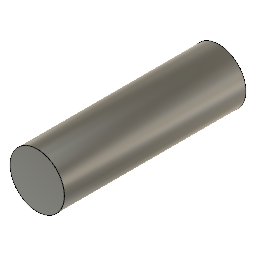
stone_holder (Autodesk Fusion 360 design; units mm, degrees)
Autodesk Fusion 360 part; units mm, degrees
sketch "Sketch1" plane through (0, 0, 0) normal (0, 0, 1) x (1, 0, 0)
  line L0 (11.2333, -2) -> (15, -2)
  line L1 (15, -2) -> (15, -102)
  line L2 (15, -102) -> (0, -102)
  line L3 (0, -102) -> (0, -10.3)
  line L4 (3.55, -6.2) -> (3.55, -10.3)
  line L5 (3.55, -10.3) -> (0, -10.3)
  line L6 (3.55, -6.2) -> (3.55, -6.0626)
  spline S0 degree 5 poles (0.0005, -6.2) (0.0004, -6.2) (0.0003, -6.2) (0.0002, -6.2) (0.0001, -6.2) (0, -6.2) knots 0.999983 0.999983 0.999983 0.999983 0.999983 0.999983 1 1 1 1 1 1
  spline S1 degree 5 poles (11.2333, -2) (11.2207, -2.1206) (11.1821, -2.3832) (11.0805, -2.7956) (10.8375, -3.3499) (10.3193, -3.992) (9.5498, -4.5477) (8.6121, -5.0047) (7.56, -5.3794) (6.3963, -5.6787) (5.3546, -5.8645) (4.4953, -5.9743) (3.8803, -6.0347) (3.558, -6.0619) (3.55, -6.0626) knots 0.274949 0.274949 0.274949 0.274949 0.274949 0.274949 0.333333 0.4 0.466667 0.533333 0.6 0.666667 0.733333 0.8 0.866667 0.86836 0.86836 0.86836 0.86836 0.86836 0.86836
  dimension "d4" = 3.55
  dimension "d5" = 4.1
  constraint horizontal L0
  constraint vertical L1
  constraint horizontal L2
  constraint vertical L3
  constraint vertical L4
  constraint horizontal L5
  measures "d4" distance of S0.end L4.start
  measures "d5" distance of S0.end L3.end
revolve "Revolve1" add sketch "Sketch1" angle 360 about axis through (0, 1.75, 0) along (0, 1, 0)
